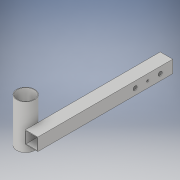
# Autodesk Inventor part: base e suporte
Saved by Autodesk Inventor 2019.4 (Build 234330000, 330)
## iProperties
Created: 2021-02-17
Part Number: base e suporte
Material: Genérico
Document SubType Name: Modeling
Designer: Lattes
Density: 1 g/cm^3
Appearance: Padrão
Author: Lattes
Autodesk Inventor part; units mm, degrees
ref_plane "YZ Plane" through (0, 0, 0) normal (1, 0, 0) x (0, 1, 0)
ref_plane "XZ Plane" through (0, 0, 0) normal (0, 1, 0) x (-1, 0, 0)
sketch "Esboço1" plane through (0, 0, 0) normal (0, 1, 0) x (-1, 0, 0)
  circle A0 centre (0, 0) radius 14.4
  circle A1 centre (0, 0) radius 13.4
  dimension "d0" = 28.8
  dimension "d1" = 1
  constraints: 2 centre point, 1 coincident
  measures "d0" diameter of A0
  measures "d1" radial gap between concentric circles of A0 A1
extrude "Extrusão1" add sketch "Esboço1" along normal blind 70
sketch "Esboço2" plane through (0, 0, 0) normal (0, -1, 0) x (1, 0, 0)
  circle A0 centre (0, 0) radius 14.4
  constraints: 1 centre point, 1 coincident
extrude "Extrusão2" add sketch "Esboço2" against normal blind 1
ref_plane "Plano de trabalho1" through (0, 0, 14.4) normal (0, 0, 1) x (1, 0, 0)
sketch "Esboço3" plane through (0, 0, 0) normal (0, 0, 1) x (1, 0, 0)
  line L0 (-14.4, 0) -> (14.4, 0) projected
  line L1 (14.4, 0) -> (14.4, 16)
  line L2 (14.4, 0) -> (14.4, 70) projected
  line L3 (14.4, 16) -> (34.4, 16)
  line L4 (14.4, 36) -> (14.4, 16)
  line L5 (34.4, 16) -> (14.4, 16)
  line L6 (14.4, 16) -> (14.4, 36)
  line L7 (14.4, 36) -> (34.4, 36)
  line L8 (34.4, 36) -> (34.4, 16)
  line L9 (34.4, 16) -> (14.4, 16)
  line L10 (14.4, 16) -> (14.4, 36)
  line L11 (15.4, 35) -> (33.4, 35)
  line L12 (33.4, 35) -> (33.4, 17)
  line L13 (15.4, 17) -> (33.4, 17)
  line L14 (15.4, 36) -> (15.4, 16)
  point P0 (0, 0)
  dimension "d7" = 16
  dimension "d8" = 20
  dimension "d11" = 1
  dimension "d12" = 1
  dimension "d13" = 1
  constraints: 26 end point, 4 parallel, 4 point on line, 3 perpendicular, 1 collinear, 1 horizontal
  measures "d7" distance of L0.end L1.end
  measures "d8" distance of L1.end L3.end
  measures "d11" distance between parallel lines of L7 L11
  measures "d12" distance between parallel lines of L3 L13
  measures "d13" distance between parallel lines of L4 L14
extrude "Extrusão3" add sketch "Esboço3" along normal blind 15 and the other way blind 200 contours L2 L7 L14 L3 | L14 L13 L12 L11 L7 L8 L3
sketch "Esboço4" plane through (0, 0, 0) normal (0, -1, 0) x (1, 0, 0)
  circle A0 centre (0, 0) radius 3
  dimension "d18" = 6
  constraints: 1 centre point, 1 coincident
  measures "d18" diameter of A0
extrude "Extrusão4" cut sketch "Esboço4" against normal blind 15
sketch "Esboço5" plane through (14.4, 16, 0) normal (-1, 0, 0) x (0, 0, 1)
  line L0 (-200, 1) -> (-200, 19) projected
  line L1 (-200, 10) -> (-180, 10)
  line L2 (-180, 10) -> (-140, 10)
  circle A0 centre (-180, 10) radius 3.25
  circle A1 centre (-140, 10) radius 3.25
  point P0 (0, -16)
  dimension "d21" = 20
  dimension "d22" = 40
  dimension "d23" = 6.5
  dimension "d24" = 6.5
  constraints: 4 end point, 2 centre point, 2 coincident, 1 horizontal, 1 midpoint, 1 point on line
  measures "d21" distance of L1.start L1.end
  measures "d22" distance of L1.end L2.end
  measures "d23" diameter of A0
  measures "d24" diameter of A1
extrude "Extrusão5" cut sketch "Esboço5" against normal blind 30
sketch "Esboço6" plane through (14.4, 16, 0) normal (-1, 0, 0) x (0, 0, 1)
  circle A0 centre (-180, 10) radius 3.25 projected
  circle A1 centre (-140, 10) radius 3.25 projected
  line L0 (-180, 10) -> (-140, 10)
  circle A2 centre (-160, 10) radius 1.75
  point P0 (0, -16)
  dimension "d27" = 3.5
  constraints: 2 end point, 1 centre point, 1 horizontal, 1 midpoint
  measures "d27" diameter of A2
extrude "Extrusão6" cut sketch "Esboço6" against normal blind 30 contours A2 L0 | L0 A2
